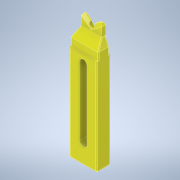
# Autodesk Inventor part: rivetclamp_2PForWheel
Saved by Autodesk Inventor 2021 (Build 250183000, 183)
## iProperties
Created: 2020-02-05
Part Number: rivetclamp_2PForWheel
Material: Generic
Document SubType Name: Modeling
Designer: shann
Density: 1 g/cm^3
Appearance: Yellow
Author: shann
Autodesk Inventor part; units mm, degrees
ref_plane "YZ Plane" through (0, 0, 0) normal (1, 0, 0) x (0, 1, 0)
ref_plane "XZ Plane" through (0, 0, 0) normal (0, 1, 0) x (-1, 0, 0)
ref_plane "XY Plane" through (0, 0, 0) normal (0, 0, 1) x (1, 0, 0)
sketch "Sketch1" plane through (0, 0, 0) normal (0, 0, 1) x (1, 0, 0)
  line L0 (0, 6.2459) -> (0, -5.08) construction
  line L1 (-9.525, 0) -> (9.525, 0) construction
  line L2 (-9.525, 3.187) -> (-9.525, -5.08)
  line L3 (-9.525, -5.08) -> (9.525, -5.08)
  line L4 (9.525, -5.08) -> (9.525, 3.187)
  line L5 (9.525, 3.187) -> (7.607, 5.7323)
  line L6 (7.607, 5.7323) -> (0, 0)
  line L7 (0, 0) -> (-7.607, 5.7323)
  line L8 (-7.607, 5.7323) -> (-9.525, 3.187)
  dimension "d1" = 19.05
  dimension "d2" = 53
  dimension "d3" = 9.525
  dimension "d23" = 5.08
  constraints: 18 end point, 4 perpendicular, 3 point on line, 2 horizontal, 2 midpoint, 1 equal length, 1 vertical, 2 other
  measures "d1" distance of L2.end L3.end
  measures "d2" angle of L0 L7
  measures "d3" distance of L6.end L7.end
  measures "d23" distance between parallel lines of L1 L3
extrude "Extrusion1" add sketch "Sketch1" along normal blind 3.81
chamfer "Chamfer1" distance 3.175 angle 22.55 2 edges at (-3.8035, 2.8661, 0) (3.8035, 2.8661, 0) measured on face at (0, -3.3867, 0)
chamfer "Chamfer2" distance 3.175 angle 22.55 2 edges at (-3.8035, 2.8661, 3.81) (3.8035, 2.8661, 3.81) measured on face at (0, -3.3867, 3.81)
sketch "Sketch2" plane through (0, 0, 0) normal (0, 0, 1) x (1, 0, 0)
  circle A0 centre (0, 0) radius 2.54
  dimension "d17" = 5.08
  constraints: 1 centre point, 1 coincident
  measures "d17" diameter of A0
extrude "Extrusion2" cut sketch "Sketch2" along normal through all both and the other way through all
sketch "Sketch3" plane through (0, 0, 0) normal (0, 0, 1) x (1, 0, 0)
  line L0 (-9.525, -5.08) -> (-12.7, -12.7)
  line L1 (-12.7, -12.7) -> (-12.7, -19.7148)
  line L2 (-12.7, -19.7148) -> (12.7, -19.7148)
  line L3 (12.7, -19.7148) -> (12.7, -12.7)
  line L4 (12.7, -12.7) -> (9.525, -5.08)
  line L5 (-9.525, -5.08) -> (9.525, -5.08) projected
  line L6 (0, 6.2459) -> (0, -5.08) construction
  line L7 (-7.607, 5.7323) -> (-9.525, 3.187) projected
  line L8 (0, 0) -> (-7.607, 5.7323) projected
  line L9 (7.607, 5.7323) -> (0, 0) projected
  line L10 (9.525, 3.187) -> (7.607, 5.7323) projected
  dimension "d20" = 7.0104
  dimension "d21" = 25.4
  constraints: 10 end point, 2 perpendicular, 1 horizontal, 2 other
  measures "d21" distance of L1.end L2.end
extrude "Extrusion3" add sketch "Sketch3" along normal blind 10.16
sketch "Sketch4" plane through (0, 0, 0) normal (1, 0, 0) x (0, 1, 0)
  line L0 (-5.08, 10.16) -> (-5.08, 3.81)
  line L1 (-5.08, 3.81) -> (-12.7, 10.16)
  line L2 (-12.7, 10.16) -> (-5.08, 10.16)
  line L3 (-5.08, 3.81) -> (3.187, 3.81) projected
  line L4 (-5.08, 0) -> (-5.08, 3.81) projected
  line L5 (-12.7, 0) -> (-12.7, 10.16) projected
  point P0 (0, 0)
  constraints: 6 end point, 1 perpendicular, 1 vertical
extrude "Extrusion4" cut sketch "Sketch4" along normal through all both and the other way through all
fillet "Fillet2" radius 0.7937 10 edges at (11.1125, -8.89, 6.985) (11.1125, -8.89, 0) (-11.1125, -8.89, 6.985) (-11.1125, -8.89, 0) (7.607, 5.7323, 1.905) (-7.607, 5.7323, 1.905) (-12.7, -16.2074, 10.16) (12.7, -16.2074, 10.16) (-12.7, -16.2074, 0) (12.7, -16.2074, 0)
sketch "Sketch10" plane through (-11.9062, -19.7148, 0) normal (0, -1, 0) x (1, 0, 0)
  line L0 (0, 10.16) -> (23.8125, 10.16) projected
  line L1 (-0.7937, 0.7937) -> (-0.7937, 9.3663) projected
  line L2 (23.8125, 0) -> (0, 0) projected
  line L3 (24.6063, 0.7937) -> (24.6063, 9.3663) projected
  line L4 (-0.7937, 11.43) -> (24.6063, 11.43)
  line L5 (24.6063, 11.43) -> (24.6062, -1.27)
  line L6 (24.6062, -1.27) -> (-0.7938, -1.27)
  line L7 (-0.7938, -1.27) -> (-0.7937, 11.43)
  line L8 (-0.7937, 11.43) -> (24.6062, -1.27) construction
  line L9 (24.6063, 11.43) -> (-0.7938, -1.27) construction
  point P0 (11.9063, 0)
  point P1 (11.9063, 5.08)
  dimension "d73" = 5.08
  dimension "d77" = 12.7
  dimension "d97" = 25.4
  dimension "d98" = 12.7
  dimension "d99" = 0
  constraints: 12 end point, 2 midpoint, 2 parallel, 1 perpendicular
  measures "d73" distance from line of point (11.906, 5.08) L0
  measures "d77" distance from line of L1 point (11.906, 5.08)
  measures "d97" distance between parallel lines of L5 L7
  measures "d98" distance between parallel lines of L4 L6
  measures "d99" angle of L0 L4
extrude "Extrusion8" add sketch "Sketch10" along normal blind 88.9
sketch "Sketch13" plane through (-12.7, -108.6148, 11.43) normal (0, 0, 1) x (1, 0, 0)
  line L0 (16.256, 81.28) -> (16.256, 17.78)
  line L1 (9.144, 17.78) -> (9.144, 81.28)
  line L2 (25.4, 88.9) -> (0, 88.9) projected
  arc A0 (16.256, 81.28) -> (9.144, 81.28) centre (12.7, 81.28) ccw
  arc A1 (9.144, 17.78) -> (16.256, 17.78) centre (12.7, 17.78) ccw
  line L3 (0, 88.9) -> (0, 0) projected
  point P0 (12.7, 108.6148)
  dimension "d110" = 7.112
  dimension "d112" = 63.5
  dimension "d113" = 3.556
  dimension "d114" = 3.556
  dimension "d115" = 7.62
  dimension "d116" = 9.144
  constraints: 4 end point, 4 point on circle, 2 centre point, 1 parallel
  measures "d110" distance between parallel lines of L0 L1
  measures "d112" distance of L1.start L1.end
  measures "d113" radius of A1
  measures "d114" radius of A0
  measures "d115" distance from line of L1.end L2
  measures "d116" distance between parallel lines of L3 L1
extrude "Extrusion10" cut sketch "Sketch13" against normal blind 25.4
fillet "Fillet11" radius 0.7937 8 edges at (12.7, -64.1648, 11.43) (-12.7, -64.1648, 11.43) (0, -108.6148, 11.43) (0, -108.6148, -1.27) (12.7, -64.1648, -1.27) (12.7, -108.6148, 5.08) (-12.7, -108.6148, 5.08) (-12.7, -64.1648, -1.27)
equation "\"RotAng\" = 0"
body "Solid1"
